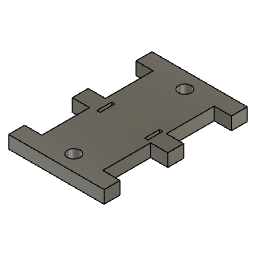
fusion 360 design (Autodesk Fusion 360 design; units mm, degrees)
Autodesk Fusion 360 part; units mm, degrees
sketch "Sketch1" plane through (0, 0, 0) normal (0, 0, 1) x (1, 0, 0)
  line L0 (0, 0) -> (-27, 0)
  line L1 (-27, 0) -> (-27, 25)
  line L2 (-27, 25) -> (0, 25)
  line L3 (0, 25) -> (0, 100)
  line L4 (0, 100) -> (-27, 100)
  line L5 (0, 0) -> (0, -75)
  line L6 (0, -75) -> (-27, -75)
  line L7 (-27, -75) -> (-27, -100)
  line L8 (-27, -100) -> (48, -100)
  line L9 (-27, 100) -> (-27, 125)
  line L10 (-27, 125) -> (48, 125)
  line L11 (48, 125) -> (123, 125)
  line L12 (123, 125) -> (123, 100)
  line L13 (123, 100) -> (96, 100)
  line L14 (96, 100) -> (96, 25)
  line L15 (96, 25) -> (123, 25)
  line L16 (123, 25) -> (123, 0)
  line L17 (123, 0) -> (96, 0)
  line L18 (96, 0) -> (96, -75)
  line L19 (96, -75) -> (123, -75)
  line L20 (123, -75) -> (123, -100)
  line L21 (123, -100) -> (48, -100)
  circle A0 centre (50, 100) radius 10
  circle A1 centre (50.5891, -75.1705) radius 10
  line L22 (9.8735, 25) -> (9.8735, 2)
  line L23 (9.8735, 2) -> (14.8735, 2)
  line L24 (14.8735, 2) -> (14.8735, 25)
  line L25 (14.8735, 25) -> (9.8735, 25)
  line L26 (89.8678, 25) -> (89.8678, 2)
  line L27 (89.8678, 2) -> (84.8678, 2)
  line L28 (84.8678, 2) -> (84.8678, 25)
  line L29 (84.8678, 25) -> (89.8678, 25)
  constraint coincident L0.start L5.start
  constraint horizontal L0
  constraint perpendicular L0 L1
  constraint perpendicular L1 L2
  constraint perpendicular L2 L3
  constraint perpendicular L3 L4
  constraint perpendicular L0 L5
  constraint perpendicular L5 L6
  constraint perpendicular L6 L7
  constraint perpendicular L7 L8
  constraint perpendicular L4 L9
  constraint perpendicular L9 L10
  constraint parallel L10 L11
  constraint perpendicular L11 L12
  constraint perpendicular L12 L13
  constraint perpendicular L13 L14
  constraint perpendicular L14 L15
  constraint perpendicular L15 L16
  constraint perpendicular L16 L17
  constraint perpendicular L17 L18
  constraint perpendicular L18 L19
  constraint perpendicular L19 L20
  constraint perpendicular L20 L21
  constraint perpendicular L2 L22
  constraint perpendicular L22 L23
  constraint perpendicular L23 L24
  constraint perpendicular L22 L25
  constraint perpendicular L15 L26
  constraint perpendicular L26 L27
  constraint perpendicular L27 L28
sketch "Sketch2" plane through (0, 0, 0) normal (0, 0, 1) x (1, 0, 0)
extrude "Extrude1" add sketch "Sketch1" along normal blind 20
